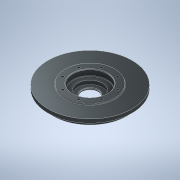
# Autodesk Inventor part: Крышка перегородки21
Saved by Autodesk Inventor 2021 (Build 250183000, 183)
## iProperties
Created: 2020-11-17
Part Number: Крышка перегородки21
Material: Чугун, серый
Document SubType Name: Modeling
Designer: Тимоха
Mass: 18482 g
Surface Area: 2478.77 cm^2
Volume: 2584.9 cm^3
Density: 7.15 g/cm^3
Appearance: Чугун серый
Author: Тимоха
Autodesk Inventor part; units mm, degrees
ref_plane "YZ Plane" through (0, 0, 0) normal (1, 0, 0) x (0, 1, 0)
ref_plane "XZ Plane" through (0, 0, 0) normal (0, 1, 0) x (-1, 0, 0)
ref_plane "XY Plane" through (0, 0, 0) normal (0, 0, 1) x (1, 0, 0)
sketch "Эскиз1" plane through (0, 0, 0) normal (0, 0, 1) x (1, 0, 0)
  line L0 (0, 0) -> (170, 0)
  line L1 (170, 0) -> (170, -15)
  line L2 (170, -15) -> (150, -15)
  line L3 (150, -15) -> (150, -35)
  line L4 (150, -35) -> (110, -35)
  line L5 (110, -35) -> (110, -42.5)
  line L6 (0, 0) -> (0, -18.1999)
  line L7 (150, -20) -> (145, -20)
  line L8 (145, -20) -> (145, -25)
  line L9 (145, -25) -> (150, -25)
  line L10 (110, -42.5) -> (32, -42.5)
  line L11 (32, -42.5) -> (32, -34.5)
  line L12 (32, -34.5) -> (50, -34.5)
  line L13 (50, -34.5) -> (50, -19.5)
  line L14 (50, -19.5) -> (70, -19.5)
  line L15 (70, -19.5) -> (70, 0)
  dimension "d0" = 170
  dimension "d1" = 15
  dimension "d2" = 20
  dimension "d3" = 20
  dimension "d4" = 40
  dimension "d5" = 7.5
  dimension "d11" = 5
  dimension "d12" = 5
  dimension "d13" = 5
  dimension "d25" = 78
  dimension "d26" = 8
  dimension "d27" = 18
  dimension "d28" = 15
  dimension "d32" = 20
  constraints: 32 end point, 11 perpendicular, 4 horizontal, 2 point on line, 1 midpoint, 1 vertical
  measures "d0" distance of L0.start L0.end
  measures "d1" distance of L0.end L1.end
  measures "d2" distance of L1.end L3.start
  measures "d3" distance of L3.start L3.end
  measures "d4" distance of L3.end L5.start
  measures "d5" distance of L5.start L5.end
  measures "d11" distance of L7.start L8.start
  measures "d12" distance of L8.start L8.end
  measures "d13" distance between parallel lines of L7 L2
  measures "d25" distance of L5.end L10.end
  measures "d26" distance of L10.end L11.end
  measures "d27" distance of L11.end L12.end
  measures "d28" distance of L12.end L13.end
  measures "d32" distance of L13.end L14.end
revolve "Вращение1" add sketch "Эскиз1" angle 360 about axis through (0, 0, 0) along (0, -1, 0) contours L0 L1 L2 L3 L7 L8 L9 L4 L5 L10 L11 L12 L13 L14 L15
chamfer "Фаска1" distance 2 angle 45 2 edges at (-32, -42.5, 0) (-32, -34.5, 0)
fillet "Сопряжение1" radius 2 1 edges at (-70, -19.5, 0)
sketch "Эскиз2" plane through (0, 0, 0) normal (0, 1, 0) x (1, 0, 0)
  circle A0 centre (0, 0) radius 100
  circle A1 centre (0, 0) radius 70 projected
  dimension "d31" = 200
  constraints: 1 centre point, 1 coincident
  measures "d31" diameter of A0
extrude "Выдавливание1" add sketch "Эскиз2" along normal blind 5
fillet "Сопряжение2" radius 2 1 edges at (-100, 0, 0)
sketch "Эскиз3" plane through (0, 5, 0) normal (0, 1, 0) x (1, 0, 0)
  circle A0 centre (0, 0) radius 70 projected
  line L0 (0, 0) -> (78.5298, 32.5281)
  line L1 (-238, 0) -> (238, 0) projected
  dimension "d36" = 85
  dimension "d37" = 22.5
  constraints: 2 end point
  measures "d36" distance of L0.start L0.end
  measures "d37" angle of L1 L0
hole "Отверстие1" at (78.5298, 5, -32.5281) direction (0, -1, 0) diameter 8 depth 15 tip angle 118 counterbore diameter 10 counterbore depth 10
pattern_circular "Круговой массив1" count 8 over 360 about axis through (0, -9.75, 0) along (0, -1, 0) of "Отверстие1"
chamfer "Фаска3" distance 2 angle 45 1 edges at (-70, 5, 0)
thread "Резьба1" size "M10x1.5" class "6H" standard "ANSI Metric M Profile" full length
thread "Резьба2" size "M10x1.5" class "6H" standard "ANSI Metric M Profile" full length
thread "Резьба3" size "M10x1.5" class "6H" standard "ANSI Metric M Profile" full length
thread "Резьба4" size "M10x1.5" class "6H" standard "ANSI Metric M Profile" full length
thread "Резьба5" size "M10x1.5" class "6H" standard "ANSI Metric M Profile" full length
thread "Резьба6" size "M10x1.5" class "6H" standard "ANSI Metric M Profile" full length
thread "Резьба7" size "M10x1.5" class "6H" standard "ANSI Metric M Profile" full length
thread "Резьба8" size "M10x1.5" class "6H" standard "ANSI Metric M Profile" full length
sketch "Эскиз4" plane through (0, -35, 0) normal (0, -1, 0) x (1, 0, 0)
  line L0 (0, 0) -> (-120.1043, -49.7488)
  line L1 (-238, 0) -> (238, 0) projected
  dimension "d67" = 130
  dimension "d68" = 22.5
  constraints: 2 end point
  measures "d67" distance of L0.start L0.end
  measures "d68" angle of L1 L0
hole "Отверстие2" at (-120.1043, -35, -49.7488) direction (0, 1, 0) diameter 8 depth 15 tip angle 118 counterbore diameter 10 counterbore depth 10
pattern_circular "Круговой массив2" count 8 over 360 about axis through (0, -41.5, 0) along (0, 1, 0) of "Отверстие2"
